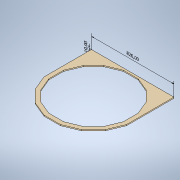
# Autodesk Inventor part: Hauptplatte
Saved by Autodesk Inventor 2020.3 (Build 243373010, 373A)
## iProperties
Created: 2021-02-11
Part Number: Hauptplatte
Material: Generisch
Document SubType Name: Modeling
Designer: Stefan
Density: 1 g/cm^3
Appearance: Pappel
Author: Stefan
Autodesk Inventor part; units mm, degrees
ref_plane "YZ Plane" through (0, 0, 0) normal (1, 0, 0) x (0, 1, 0)
ref_plane "XZ Plane" through (0, 0, 0) normal (0, 1, 0) x (-1, 0, 0)
ref_plane "XY Plane" through (0, 0, 0) normal (0, 0, 1) x (1, 0, 0)
sketch "Skizze2" plane through (0, 0, 0) normal (0, 1, 0) x (-1, 0, 0)
  line L0 (326.749, 800) -> (176.0567, 737.5812)
  line L1 (176.0567, 737.5812) -> (60.7218, 622.2463)
  line L2 (60.7218, 622.2463) -> (-1.697, 471.5541)
  line L3 (-1.697, 471.5541) -> (-1.697, 0)
  line L4 (-1.697, 0) -> (0, 0)
  line L5 (0, 0) -> (816.6061, 0)
  line L6 (816.6061, 0) -> (818.303, 0)
  line L7 (818.303, 0) -> (818.303, 471.5541)
  line L8 (818.303, 471.5541) -> (755.8842, 622.2463)
  line L9 (755.8842, 622.2463) -> (640.5494, 737.5812)
  line L10 (640.5494, 737.5812) -> (489.8571, 800)
  line L11 (489.8571, 800) -> (326.749, 800)
  line L12 (617.8912, 76.3291) -> (481.9006, 20)
  line L13 (481.9006, 20) -> (334.7055, 20)
  line L14 (334.7055, 20) -> (198.7149, 76.3291)
  line L15 (198.7149, 76.3291) -> (94.6322, 180.4118)
  line L16 (94.6322, 180.4118) -> (38.303, 316.4024)
  line L17 (38.303, 316.4024) -> (38.303, 463.5976)
  line L18 (38.303, 463.5976) -> (94.6322, 599.5882)
  line L19 (94.6322, 599.5882) -> (198.7149, 703.6709)
  line L20 (198.7149, 703.6709) -> (334.7055, 760)
  line L21 (334.7055, 760) -> (481.9006, 760)
  line L22 (481.9006, 760) -> (617.8912, 703.6709)
  line L23 (617.8912, 703.6709) -> (721.9739, 599.5882)
  line L24 (721.9739, 599.5882) -> (778.303, 463.5976)
  line L25 (778.303, 463.5976) -> (778.303, 316.4024)
  line L26 (778.303, 316.4024) -> (721.9739, 180.4118)
  line L27 (721.9739, 180.4118) -> (617.8912, 76.3291)
  point P0 (481.9006, 20)
  dimension "d89" = 157.5
  dimension "d90" = 22.5
  dimension "d91" = 135
  dimension "d92" = 90
  dimension "d93" = 90
  dimension "d94" = 40
  dimension "d95" = 780
  dimension "d96" = 820
  dimension "d97" = 800
  dimension "d98" = 760
  dimension "d99" = 20
  dimension "d100" = 40
  dimension "d101" = 780
  dimension "d102" = 740
  dimension "d103" = 780
  dimension "d104" = 40
  dimension "d105" = 780
  dimension "d106" = 740
  dimension "d107" = 780
  dimension "d108" = 40
  dimension "d109" = 780
  dimension "d110" = 740
  dimension "d111" = 780
  dimension "d112" = 818.303
  dimension "d113" = 0
  dimension "d114" = 936.4693
  dimension "d115" = 597.9763
  dimension "d116" = 974.4855
  dimension "d117" = 382.9422
  dimension "d118" = 926.5638
  dimension "d119" = 165.9378
  dimension "d120" = 0
  dimension "d121" = 0
  dimension "d122" = 0
  dimension "d123" = 471.5541
  dimension "d124" = 0
  dimension "d125" = 0
  dimension "d126" = 1.697
  dimension "d127" = 1.697
  dimension "d128" = 40
  dimension "d129" = 463.5976
  dimension "d130" = 40
  dimension "d131" = 316.4024
  dimension "d132" = 62.4188
  dimension "d133" = 62.4188
  dimension "d134" = 96.3291
  dimension "d135" = 96.3291
  dimension "d136" = 96.3291
  dimension "d137" = 96.3291
  dimension "d138" = 177.7537
  dimension "d139" = 177.7537
  dimension "d140" = 200.4118
  dimension "d141" = 200.4118
  dimension "d142" = 200.4118
  dimension "d143" = 200.4118
  dimension "d144" = 328.4459
  dimension "d145" = 328.4459
  dimension "d146" = 336.4024
  dimension "d147" = 336.4024
  dimension "d148" = 336.4024
  dimension "d149" = 336.4024
  dimension "d150" = 483.5976
  dimension "d151" = 483.5976
  dimension "d152" = 483.5976
  constraints: 56 end point, 18 parallel, 3 perpendicular, 1 horizontal, 1 vertical
  measures "d89" angle of L7 L8
  measures "d90" angle of L7 L26
  measures "d91" angle of L7 L9
  measures "d92" angle of L7 L5
  measures "d93" angle of L7 L4
  measures "d94" distance between parallel lines of L7 L25
  measures "d95" distance between parallel lines of L7 L17
  measures "d96" distance between parallel lines of L7 L3
  measures "d97" distance between parallel lines of L6 L11
  measures "d98" distance between parallel lines of L6 L21
  measures "d99" distance between parallel lines of L6 L13
  measures "d100" distance between parallel lines of L8 L24
  measures "d101" distance between parallel lines of L8 L16
  measures "d102" distance between parallel lines of L18 L26
  measures "d103" distance between parallel lines of L2 L26
  measures "d104" distance between parallel lines of L9 L23
  measures "d105" distance between parallel lines of L9 L15
  measures "d106" distance between parallel lines of L19 L27
  measures "d107" distance between parallel lines of L1 L27
  measures "d108" distance between parallel lines of L10 L22
  measures "d109" distance between parallel lines of L10 L14
  measures "d110" distance between parallel lines of L12 L20
  measures "d111" distance between parallel lines of L12 L0
  measures "d112" distance from line of point (0, 0) L7
  measures "d113" distance from line of point (0, 0) L6
  measures "d114" distance from line of point (0, 0) L8
  measures "d115" distance from line of point (0, 0) L26
  measures "d116" distance from line of point (0, 0) L9
  measures "d117" distance from line of point (0, 0) L27
  measures "d118" distance from line of point (0, 0) L10
  measures "d119" distance from line of point (0, 0) L12
  measures "d120" distance from line of point (0, 0) L5
  measures "d121" distance from line of point (0, 0) L4
  measures "d122" distance from line of L8.start L7
  measures "d123" distance from line of L7.end L6
  measures "d124" distance from line of L7.start L6
  measures "d125" distance from line of L6.end L7
  measures "d126" distance from line of L5.end L7
  measures "d127" distance from line of L6.start L7
  measures "d128" distance from line of L24.end L7
  measures "d129" distance from line of L25.start L6
  measures "d130" distance from line of L26.start L7
  measures "d131" distance from line of L25.end L6
  measures "d132" distance from line of L8.end L7
  measures "d133" distance from line of L9.start L7
  measures "d134" distance from line of L24.start L7
  measures "d135" distance from line of L23.end L7
  measures "d136" distance from line of L27.start L7
  measures "d137" distance from line of L26.end L7
  measures "d138" distance from line of L9.end L7
  measures "d139" distance from line of L10.start L7
  measures "d140" distance from line of L23.start L7
  measures "d141" distance from line of L22.end L7
  measures "d142" distance from line of L12.start L7
  measures "d143" distance from line of L27.end L7
  measures "d144" distance from line of L10.end L7
  measures "d145" distance from line of L11.start L7
  measures "d146" distance from line of L22.start L7
  measures "d147" distance from line of L21.end L7
  measures "d148" distance from line of L12.end L7
  measures "d149" distance from line of L13.start L7
  measures "d150" distance from line of L20.end L7
  measures "d151" distance from line of L21.start L7
  measures "d152" distance from line of L14.start L7
extrude "Extrusion1" add sketch "Skizze2" along normal blind 10
